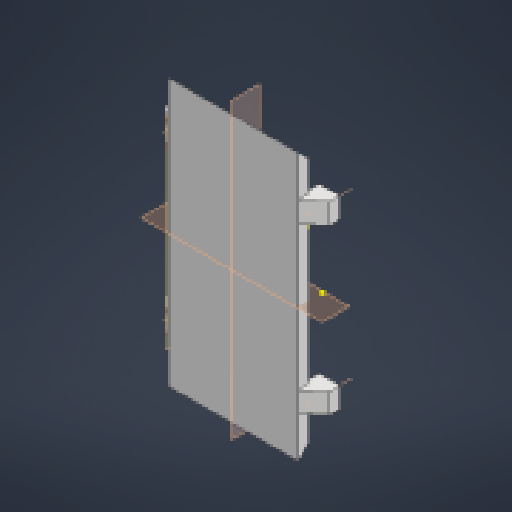
# Autodesk Inventor part: Krone_interface
Saved by Autodesk Inventor 2023.4 (Build 274418000, 418)
## iProperties
Created: 2025-10-22
Part Number: Krone_interface
Material: Generic
Document SubType Name: Modeling
Designer: Malthe Sennels
Density: 1 g/cm^3
Appearance: Default
Author: Malthe Sennels
Autodesk Inventor part; units mm, degrees
ref_plane "XZ Plane" through (0, 0, 0) normal (0, 1, 0) x (-1, 0, 0)
ref_plane "XY Plane" through (0, 0, 0) normal (0, 0, 1) x (1, 0, 0)
ref_plane "Work Plane1" through (35, 40, 0) normal (0, 1, 0) x (0, 0, -1)
ref_plane "Work Plane2" through (35, -40, 0) normal (0, 1, 0) x (0, 0, -1)
sketch "Sketch1" plane through (35, 40, 0) normal (0, 1, 0) x (0, 0, -1)
  line L0 (0, -1.75) -> (0, 1.75) projected
  line L1 (0, 68.25) -> (0, 71.75) projected
  line L2 (0, -5) -> (-5, -5)
  line L3 (-5, -5) -> (-5, 5)
  line L4 (-5, 5) -> (0, 5)
  line L5 (0, 5) -> (0, -5)
  line L6 (3, -1.75) -> (0, -1.75)
  line L7 (3, 1.75) -> (0, 1.75)
  line L8 (-54.9316, 0) -> (12.6553, 0) projected
  line L9 (0, 35) -> (-45.2764, 35) construction
  line L10 (-5, 5) -> (-6, 8.7321)
  line L11 (-6, 8.7321) -> (-6, 35)
  line L12 (-12, 35) -> (-12, 3.3423)
  line L13 (-12, 3.3423) -> (-5, -5)
  line L14 (0, 71.75) -> (0, 68.25)
  line L15 (0, 75) -> (-5, 75)
  line L16 (-5, 75) -> (-5, 65)
  line L17 (-5, 65) -> (0, 65)
  line L18 (0, 65) -> (0, 75)
  line L19 (-5, 65) -> (-6, 61.2679)
  line L20 (-6, 61.2679) -> (-6, 35)
  line L21 (-12, 35) -> (-12, 66.6577)
  line L22 (-12, 66.6577) -> (-5, 75)
  point P0 (0, 75)
  dimension "d0" = 5
  dimension "d1" = 5
  dimension "d2" = 105
  dimension "d3" = 40
  dimension "d4" = 6
  dimension "d5" = 12
  constraints: 40 end point, 6 symmetric about line, 4 horizontal, 2 parallel, 2 perpendicular, 2 point on line, 1 vertical, 4 other
  measures "d0" distance between parallel lines of L8 L4
  measures "d1" distance between parallel lines of L3 L5
  measures "d2" angle of L4 L10
  measures "d3" angle of L3 L13
  measures "d4" distance between parallel lines of L12 L11
  measures "d5" distance from line of L4.end L12
extrude "Extrusion1" add sketch "Sketch1" along normal mid plane 10
ref_plane "Work Plane3" through (35, 0, 0) normal (0, 1, 0) x (0, 0, -1)
mirror "Mirror1" about plane through (35, 0, 0) normal (0, 1, 0) of "Extrusion1"
ref_plane "Work Plane4" through (-31.6577, 40, 12) normal (-1, 0, 0) x (0, 1, 0)
sketch "Sketch2" plane through (-31.6577, 40, 12) normal (-1, 0, 0) x (0, 1, 0)
  line L0 (-5, 0) -> (5, 0) projected
  line L1 (5, 7) -> (5, 0) construction
  line L2 (-5, 7) -> (5, 7) construction
  line L3 (-5, 0) -> (-5, 7) construction
  line L4 (-75, 0) -> (-85, 0) projected
  line L5 (-75, 0) -> (-75, 7) construction
  line L6 (-75, 7) -> (-85, 7) construction
  line L7 (-85, 7) -> (-85, 0) construction
  line L8 (-40, 0) -> (-100, 0)
  line L9 (-100, 0) -> (-100, 5) construction
  line L10 (-100, 5) -> (-40, 5)
  line L11 (-40, 5) -> (-40, 0) construction
  line L12 (-100, 5) -> (-105, 0)
  line L13 (-100, 5) -> (-92.9289, 5) construction
  line L14 (-105, 0) -> (-100, 0)
  line L15 (-40, 0) -> (20, 0)
  line L16 (20, 0) -> (20, 5) construction
  line L17 (20, 5) -> (-40, 5)
  line L18 (20, 5) -> (25, 0)
  line L19 (25, 0) -> (20, 0)
  point P0 (-40, 12)
  dimension "d9" = 5
  dimension "d10" = 135
  dimension "d11" = 65
  constraints: 24 end point, 3 horizontal, 3 symmetric about line, 2 parallel, 2 point on line, 1 equal length, 1 perpendicular
  measures "d9" distance of L8.end L9.end
  measures "d10" angle of L12 L13
  measures "d11" distance of L12.end L8.start
extrude "Extrusion2" add sketch "Sketch2" against normal up to surface (63.3154 mm away)
sketch "Sketch3" plane through (31.6577, 45, 12) normal (1, 0, 0) x (0, 0, -1)
  point P0 (12, -45)
  point P1 (5, -10)
ref_plane "Work Plane5" through (15, 0, 0) normal (1, 0, 0) x (0, 1, 0)
sketch "Sketch4" plane through (15, 0, 0) normal (1, 0, 0) x (0, 1, 0)
  line L0 (65, 12) -> (60, 7) projected
  line L1 (65, 12) -> (65, 37)
  line L2 (65, 37) -> (60, 37)
  line L3 (60, 37) -> (60, 12)
  line L4 (45, 12) -> (65, 12) projected
  line L5 (45, 5) -> (45, 12) projected
  line L6 (35, 12) -> (35, 5) projected
  line L7 (45, 12) -> (35, 12)
  line L8 (35, 12) -> (35, 19.5)
  line L9 (37.5, 22) -> (42.5, 22)
  line L10 (45, 19.5) -> (45, 12)
  circle A0 centre (40, 17) radius 2.25
  arc A1 (45, 19.5) -> (42.5, 22) centre (42.5, 19.5) ccw
  arc A2 (37.5, 22) -> (35, 19.5) centre (37.5, 19.5) ccw
  line L11 (0, 12) -> (0, 44.368)
  line L12 (-65, 12) -> (-65, 37)
  line L13 (-65, 37) -> (-60, 37)
  line L14 (-60, 37) -> (-60, 12)
  line L15 (-45, 12) -> (-65, 12)
  line L16 (-45, 12) -> (-35, 12)
  line L17 (-35, 12) -> (-35, 19.5)
  line L18 (-37.5, 22) -> (-42.5, 22)
  line L19 (-45, 19.5) -> (-45, 12)
  circle A3 centre (-40, 17) radius 2.25
  arc A4 (-42.5, 22) -> (-45, 19.5) centre (-42.5, 19.5) ccw
  arc A5 (-35, 19.5) -> (-37.5, 22) centre (-37.5, 19.5) ccw
  point P0 (0, 0)
  point P1 (62.5, 37)
  point P2 (35, 22)
  point P3 (40, 22)
  point P4 (-62.5, 37)
  point P5 (-35, 22)
  point P6 (-40, 22)
  dimension "d15" = 5
  dimension "d16" = 25
  dimension "d17" = 10
  dimension "d18" = 4.5
  dimension "d19" = 5
  dimension "d20" = 5
  dimension "d21" = 2.5
  constraints: 32 end point, 17 symmetric about line, 8 point on circle, 8 point on line, 6 centre point, 4 tangent, 2 horizontal, 2 midpoint, 2 parallel, 2 perpendicular, 2 vertical, 1 equal radius, 3 other
  measures "d15" distance between parallel lines of L1 L3
  measures "d16" distance from line of point (62.5, 37) L4
  measures "d17" distance of L7.end point (35, 22)
  measures "d18" diameter of A0
  measures "d19" distance of point (40, 22) A0.centre
  measures "d20" distance from line of L10 A0.centre
  measures "d21" radius of A1
extrude "Extrusion3" add sketch "Sketch4" against normal blind 10
sketch "Sketch5" plane through (-31.6577, -35, 12) normal (0, 0, 1) x (1, 0, 0)
  line L0 (46.6577, 100) -> (46.6577, 95) projected
  line L1 (46.6577, 100) -> (49.8577, 100)
  line L2 (49.8577, 100) -> (49.8577, 97)
  line L3 (49.8577, 97) -> (46.6577, 97)
  line L4 (46.6577, 97) -> (46.6577, 100)
  line L5 (0, 95) -> (63.3154, 95) projected
  line L6 (49.8577, 100) -> (52.8577, 100)
  line L7 (52.8577, 100) -> (52.8577, 95)
  line L8 (52.8577, 95) -> (49.8577, 95)
  line L9 (49.8577, 95) -> (49.8577, 100)
  line L10 (63.3154, 35) -> (0, 35)
  line L11 (46.6577, -30) -> (46.6577, -25)
  line L12 (46.6577, -30) -> (49.8577, -30)
  line L13 (49.8577, -30) -> (49.8577, -27)
  line L14 (49.8577, -27) -> (46.6577, -27)
  line L15 (46.6577, -27) -> (46.6577, -30)
  line L16 (49.8577, -30) -> (52.8577, -30)
  line L17 (52.8577, -30) -> (52.8577, -25)
  line L18 (52.8577, -25) -> (49.8577, -25)
  line L19 (49.8577, -25) -> (49.8577, -30)
  point P0 (31.6577, 35)
  dimension "d24" = 3.2
  dimension "d25" = 3
  dimension "d26" = 3
  constraints: 36 end point, 8 symmetric about line, 4 parallel, 3 horizontal, 2 perpendicular, 1 midpoint, 1 point on line
  measures "d24" distance of L2.end L3.end
  measures "d25" distance of L1.end L2.end
  measures "d26" distance of L7.end L8.end
extrude "Extrusion4" add sketch "Sketch5" along normal up to surface (25 mm away) contours L1 L2 L3 L0 | L6 L7 L5 L9 L2 | L11 L14 L13 L12 | L13 L19 L18 L17 L16
sketch "Sketch6" plane through (5, -60, 37) normal (0, 0, 1) x (1, 0, 0)
  line L0 (16.2, 0) -> (16.2, -5) projected
  line L1 (0, -5) -> (16.2, -5) projected
  line L2 (16.2, 0) -> (7, 0)
  line L3 (7, 0) -> (7, -5)
  line L4 (7, -5) -> (16.2, -5)
  line L5 (16.2, -5) -> (16.2, 0)
  line L6 (10, 0) -> (10, -2) projected
  line L7 (10, 0) -> (10, -2) projected
  line L8 (10, 0) -> (0, 0) projected
  line L9 (0, -5) -> (0, 0) projected
  line L10 (16.2, -5) -> (0, -5) projected
  line L11 (16.2, 0) -> (16.2, -5) projected
  line L12 (13.2, 0) -> (16.2, 0) projected
  line L13 (13.2, -2) -> (13.2, 0) projected
  line L14 (10, -2) -> (13.2, -2) projected
  line L15 (0, 125) -> (16.2, 125) projected
  line L16 (0, 120) -> (0, 125) projected
  line L17 (10, 120) -> (0, 120) projected
  line L18 (10, 122) -> (10, 120) projected
  line L19 (13.2, 122) -> (10, 122) projected
  line L20 (13.2, 120) -> (13.2, 122) projected
  line L21 (16.2, 120) -> (13.2, 120) projected
  line L22 (16.2, 125) -> (16.2, 120) projected
  line L23 (16.2, 120) -> (13.2, 120) projected
  line L24 (0, 125) -> (16.2, 125) projected
  line L25 (16.2, 120) -> (7, 120)
  line L26 (7, 120) -> (7, 125)
  line L27 (7, 125) -> (16.2, 125)
  line L28 (16.2, 125) -> (16.2, 120)
  point P0 (-5, 60)
  point P1 (7, -2.5)
  point P2 (10, 121)
  point P3 (7, 0)
  dimension "d29" = 3
  dimension "d30" = 3
  constraints: 16 end point, 4 parallel, 2 horizontal, 2 midpoint, 2 perpendicular, 2 point on line
  measures "d29" distance from line of L6 point (7, -2.5)
  measures "d30" distance from line of point (10, 121) L26
extrude "Extrusion5" cut sketch "Sketch6" against normal up to surface (25 mm away) contours L1 L9 L8 L3 | L15 L26 L17 L16
mirror "Mirror2" about plane through (0, 0, 0) normal (1, 0, 0) of "Extrusion5", "Extrusion4", "Extrusion3"
chamfer "Chamfer1" distance 10 angle 45 8 edges at (-19.7, 60, 12) (-13.5, 60, 12) (13.5, 60, 12) (19.7, 60, 12) (-19.7, -60, 12) (-13.5, -60, 12) (13.5, -60, 12) (19.7, -60, 12)
sketch "Sketch7" plane through (-21.2, 60, 37) normal (-1, 0, 0) x (0, 0, 1)
  line L0 (0, 0) -> (0, 5) projected
  line L1 (0, 0) -> (-25, -53.6127)
  line L2 (-25, -95) -> (-25, -25) projected
  line L3 (-15, 0) -> (0, 0) projected
  line L4 (-6.6203, 0) -> (-25, -39.4155)
  line L5 (-25, -25) -> (-25, -95) projected
  line L6 (-25, -60) -> (1.6429, -60)
  line L7 (0, -120) -> (-25, -66.3873)
  line L8 (-6.6203, -120) -> (-25, -80.5845)
  line L9 (-15, -120) -> (0, -120) projected
  point P0 (-37, -60)
  dimension "d36" = 6
  dimension "d37" = 65
  constraints: 10 end point, 4 symmetric about line, 3 point on line, 1 horizontal, 1 midpoint, 1 parallel
  measures "d36" distance between parallel lines of L1 L4
  measures "d37" angle of L3 L1
extrude "Extrusion6" add sketch "Sketch7" against normal blind 3
sketch "Sketch8" plane through (-31.6577, -35, 12) normal (0, 0, 1) x (1, 0, 0)
  line L0 (63.3154, 70) -> (63.3154, 80) projected
  line L1 (63.3154, 0) -> (63.3154, -10) projected
  line L2 (0, 0) -> (0, -10) projected
  line L3 (0, 70) -> (0, 80) projected
  line L4 (0, 80) -> (0, 100) projected
  line L5 (52.8577, -30) -> (63.3154, -30) projected
  line L6 (0, 100) -> (63.3154, 100)
  line L7 (63.3154, 100) -> (63.3154, -30)
  line L8 (63.3154, -30) -> (0, -30)
  line L9 (0, -30) -> (0, 100)
  line L10 (63.3154, 70) -> (63.3154, 0) projected
  line L11 (63.3154, 0) -> (0, 0)
  line L12 (0, 0) -> (0, -10)
  line L13 (0, -10) -> (63.3154, -10)
  line L14 (63.3154, -10) -> (63.3154, 0)
  line L15 (0, -30) -> (10.4577, -30) projected
  line L16 (19.6577, 95) -> (19.6577, 100) projected
  line L17 (10.4577, -30) -> (19.6577, -30)
  line L18 (19.6577, -30) -> (19.6577, 100)
  line L19 (19.6577, 100) -> (10.4577, 100)
  line L20 (10.4577, 100) -> (10.4577, -30)
  line L21 (19.6577, 100) -> (43.6577, 100) projected
  line L22 (43.6577, 100) -> (52.8577, 100)
  line L23 (52.8577, 100) -> (52.8577, -30)
  line L24 (52.8577, -30) -> (43.6577, -30)
  line L25 (43.6577, -30) -> (43.6577, 100)
  line L26 (0, 80) -> (63.3154, 80) projected
  line L27 (63.3154, 80) -> (0, 80)
  line L28 (0, 80) -> (0, 70)
  line L29 (0, 70) -> (63.3154, 70)
  line L30 (63.3154, 70) -> (63.3154, 80)
  line L31 (0, 70) -> (-8.3423, 70) projected
  line L32 (0, 70) -> (10.4577, 59.5423)
  line L33 (10.4577, 95) -> (10.4577, 55.5845) projected
  line L34 (0, 70) -> (14.7895, 70) construction
  line L35 (10.4577, 35) -> (52.8577, 35) construction
  line L36 (31.6577, 100) -> (31.6577, -30) construction
  line L37 (19.6577, -30) -> (43.6577, -30) projected
  line L38 (0, 0) -> (10.4577, 10.4577)
  line L39 (63.3154, 70) -> (52.8577, 59.5423)
  line L40 (63.3154, 0) -> (52.8577, 10.4577)
  line L41 (63.3154, -10) -> (52.8577, -10)
  line L42 (52.8577, -10) -> (52.8577, -30)
  line L43 (52.8577, -30) -> (63.3154, -30)
  line L44 (63.3154, -30) -> (63.3154, -10)
  point P0 (31.6577, 35)
  point P1 (52.8577, 80)
  point P2 (19.6577, 80)
  point P3 (43.6577, 80)
  point P4 (10.4577, 80)
  point P5 (10.4577, 10.4577)
  point P6 (10.4577, 59.5423)
  point P7 (43.6577, 70)
  point P8 (19.6577, 70)
  point P9 (19.6577, 0)
  point P10 (43.6577, 0)
  point P11 (43.6577, -30)
  point P12 (43.6577, -10)
  point P13 (19.6577, -10)
  point P14 (19.6577, -30)
  point P15 (10.4577, -10)
  dimension "d40" = 45
  constraints: 62 end point, 12 parallel, 7 horizontal, 6 perpendicular, 4 midpoint, 4 symmetric about line, 1 equal length, 1 point on line
  measures "d40" angle of L32 L34
extrude "Extrusion7" cut sketch "Sketch8" against normal up to surface (5 mm away) contours L7 L40 L23 L39 | L26 L23 L6 L7 | L7 L5 L23 L13 | L25 L11 L18 L29 | L26 L18 L16 L6 L25 | L25 L8 L18 L13 | L26 L4 L6 L20 | L20 L38 L9 L32 | L20 L8 L9 L13
sketch "Sketch9" plane through (-21.2, -65, 37) normal (0, -1, 0) x (1, 0, 0)
  line L0 (33.2, -25) -> (33.2, 0) projected
  line L1 (9.2, -25) -> (9.2, 0) projected
  line L2 (33.2, 0) -> (9.2, 0)
  line L3 (33.2, -6.5) -> (27.2, -12.5)
  line L4 (27.2, -12.5) -> (33.2, -18.5)
  line L5 (33.2, -25) -> (9.2, -25)
  line L6 (21.2, 0) -> (21.2, -25) construction
  line L7 (26.2, -25) -> (16.2, -25) projected
  line L8 (21.2, -12.5) -> (33.2, -12.5) construction
  line L9 (9.2, -6.5) -> (15.2, -12.5)
  line L10 (15.2, -12.5) -> (9.2, -18.5)
  line L11 (33.2, 0) -> (21.2, -12)
  line L12 (9.2, 0) -> (21.2, -12)
  line L13 (33.2, -25) -> (21.2, -13)
  line L14 (9.2, -25) -> (21.2, -13)
  line L15 (24.7, -8.5) -> (17.7, -8.5)
  line L16 (24.7, -16.5) -> (17.7, -16.5)
  point P0 (21.2, -37)
  point P1 (9.2, -6.5)
  point P2 (9.2, -18.5)
  point P3 (17.7, -16.5)
  point P4 (33.2, 0)
  dimension "d43" = 90
  dimension "d44" = 45
  dimension "d45" = 6
  dimension "d48" = 4
  constraints: 28 end point, 8 symmetric about line, 7 point on line, 5 midpoint, 3 horizontal, 1 parallel, 1 perpendicular
  measures "d43" angle of L3 L4
  measures "d44" angle of L3 L8
  measures "d45" distance from line of L6 L3.end
  measures "d48" distance between parallel lines of L15 L8
extrude "Extrusion8" add sketch "Sketch9" against normal blind 3 contours L13 L14 L1 L10 L9 L12 L11 L0 L3 L4 | L16 L14 L13 | L11 L12 L15
mirror "Mirror3" about plane through (35, 0, 0) normal (0, 1, 0) of "Extrusion8"
mirror "Mirror4" about plane through (0, 0, 0) normal (1, 0, 0) of "Extrusion6"
body "Solid1"
